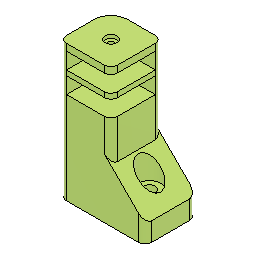
Idler Mount v18 (Autodesk Fusion 360 design; units mm, degrees)
Autodesk Fusion 360 part; units mm, degrees
note: some values were not read from the file. Chosen so that the rebuilt part matches the saved one: which face or edge a step refers to; which pieces of a blend or face edit are solid. Set by a fixed rule: which sketch regions a step uses.
box "BoxPrimitive1" add length 30 width 30 height 51.95 placed x (0, 0, 1) y (1, 0, 0) z (0, 1, 0) at (-10, 0, 0) makes body 1
box "BoxPrimitive2" add length 30 width 30 height 25.975 placed x (0, 0, 1) y (1, 0, 0) z (0, 1, 0) at (10, 0, 0) bodies 1
chamfer "Chamfer1" distance 20 angle 45 1 edges at (40, 25.975, 15) on bodies 1
sketch "Sketch3" plane through (0, 0, 0) normal (0, -1, 0) x (1, 0, 0)
  line L0 (40, 30) -> (-10, 30)
  line L1 (-10, 30) -> (-10, 0)
  line L2 (-10, 0) -> (40, 0)
  line L3 (40, 0) -> (40, 30)
  line L4 (0, 0) -> (20, 0) construction
  line L5 (19.9999, 30) -> (40, 30) construction
  line L6 (40, 30) -> (40, 0) construction
  line L7 (20, 0) -> (40, 0) construction
  line L8 (-10, 0) -> (-10, 30)
  line L9 (-10, 30) -> (40, 30)
  line L10 (-10, 0) -> (40, 0)
  line L11 (15, 30) -> (15, 0) construction
  line L12 (15, 0) -> (40, 30) construction
  line L13 (15, 30) -> (40, 0) construction
  circle A0 centre (27.5, 15) radius 3.5
move_body "Move1" bodies 1 to x (1, 0, 0) y (0, 1, 0) z (0, 0, 1) at (0, 5, 0)
extrude "Extrude1" add 1 faces at (6.6667, 5, 20) along direction (0, -1, 0) blind 5 on bodies 1 bodies 1
extrude "Extrude2" cut 1 faces at (10, 56.95, 10) along direction (0, -1, 0) blind 5 on bodies 1 bodies 1
fillet "Fillet1" radius 10 1 edges at (-10, 25.975, 0) on bodies 1
sketch "Sketch6" plane through (0, 51.95, 0) normal (0, 1, 0) x (-1, 0, 0)
  arc A0 (0, 0) -> (10, 10) centre (0, 10) ccw
  line L0 (10, 10) -> (10, 30)
  line L1 (10, 30) -> (-20, 30)
  line L2 (-20, 30) -> (-20, 0)
  line L3 (-20, 0) -> (0, 0)
  line L4 (-20, 0) -> (0, 0)
  line L5 (10, 30) -> (10, 10)
  line L6 (-20, 0) -> (-20, 30)
  line L7 (-20, 30) -> (10, 30)
  arc A1 (0, 0) -> (10, 10) centre (0, 10) ccw
  line L8 (10, 10) -> (10, 0)
  line L9 (10, 0) -> (0, 0)
  line L10 (10, 0) -> (-20, 30) construction
  line L11 (10, 30) -> (-20, 0) construction
  circle A2 centre (-5, 15) radius 1.5
  circle A3 centre (-5, 15) radius 11
  circle A4 centre (-5, 15) radius 2
  line L12 (-5, 15) -> (10, 15) construction
  line L13 (-5, 15) -> (-20, 15) construction
  line L14 (6, 15) -> (6, 30)
  line L15 (-5, 15) -> (-5, 4)
  line L16 (-5, 4) -> (-20, 4)
  line L17 (-16, 26) -> (-16, 30)
  line L18 (-16, 26) -> (-20, 26)
  line L19 (-16, 15) -> (-16, 26) construction
  line L20 (-5, 26) -> (-16, 26) construction
  dimension "d41" = 22
  measures "d41" diameter of A3
extrude "Extrude4" add 1 faces at (13.3333, 51.95, 10) along direction (0, 1, 0) blind 9 separate body on bodies 1 makes body 2
extrude "Extrude5" add 1 faces at (13.3333, 60.95, 10) along direction (0, 1, 0) blind 3 separate body on bodies 2 makes body 3
extrude "Extrude6" add 1 faces at (13.3333, 63.95, 10) along direction (0, 1, 0) blind 9 separate body on bodies 3 makes body 4
extrude "Extrude7" add 1 faces at (13.3333, 72.95, 10) along direction (0, 1, 0) blind 3 separate body on bodies 4 makes body 5
extrude "Extrude11" cut sketch "Sketch3" against normal blind 50 contours A0 bodies 1
sketch "Sketch10" plane through (0, 0, 0) normal (0, -1, 0) x (1, 0, 0)
  circle A0 centre (27.5, 15) radius 3.5
  arc A1 (-10, 10) -> (0, 0) centre (0, 10) ccw
  line L0 (0, 0) -> (40, 0)
  line L1 (40, 0) -> (40, 30)
  line L2 (40, 30) -> (-10, 30)
  line L3 (-10, 30) -> (-10, 10)
ref_plane "WorkPlane1" through (15, 15, 15) normal (0, -1, 0) x (1, 0, 0)
sketch "Sketch11" plane through (15, 15, 15) normal (0, -1, 0) x (1, 0, 0)
  circle A0 centre (12.5, 0) radius 3.5
  circle A1 centre (12.5, 0) radius 3.5
  line L0 (12.5, 0) -> (12.476, -3.4999)
cylinder "CylinderPrimitive4" cut diameter 13 height -21 placed x (1, 0, 0) y (0, 0, 1) z (0, -1, 0) at (27.5, 15, 15) bodies 1
extrude "Extrude12" cut sketch "Sketch6" along normal blind 38 contours A2 bodies 3 5
extrude "Extrude13" cut sketch "Sketch6" along normal blind 21 contours L1 L2 L6 L7 A3 L14 L16 L17 L18 | L1 L2 L6 L7 L17 L18 | A3 | A2 | A4 bodies 2 4
extrude "Extrude14" add sketch "Sketch6" along normal blind 24 contours L1 L2 L6 L7 L17 L18 bodies 3 2 1 5
sketch "Sketch12" plane through (0, 75.95, 0) normal (0, 1, 0) x (-1, 0, 0)
  circle A0 centre (-5, 15) radius 1.5
  line L0 (10, 30) -> (-20, 30)
  line L1 (-20, 30) -> (-20, 0)
  line L2 (-20, 0) -> (0, 0)
  arc A1 (0, 0) -> (10, 10) centre (0, 10) ccw
  line L3 (10, 10) -> (10, 30)
  line L4 (10, 30) -> (-20, 0) construction
  line L5 (-20, 30) -> (10, 0) construction
  line L6 (10, 0) -> (10, 30) construction
  line L7 (10, 0) -> (-20, 0) construction
  line L8 (-20, 0) -> (-20, 30) construction
  line L9 (-20, 30) -> (10, 30) construction
  circle A2 centre (-5, 15) radius 3.5
extrude "Extrude15" cut sketch "Sketch12" against normal blind 2 contours A2 bodies 3
extrude "Extrude16" add 1 faces at (4.9128, 75.95, 26.1634) along direction (0, 1, 0) blind 1 on bodies 3 bodies 3
extrude "Extrude17" add 1 faces at (2.1853, 73.95, 14.7516) along direction (0, 1, 0) blind 1 on bodies 3 bodies 3
extrude "Extrude18" cut sketch "Sketch6" against normal blind 8 contours A2 bodies 3
sketch "Sketch13" plane through (0, 63.95, 0) normal (0, 1, 0) x (-1, 0, 0)
  line L0 (-16, 26) -> (-20, 26)
  line L1 (-20, 26) -> (-20, 0)
  line L2 (-20, 0) -> (0, 0)
  arc A0 (0, 0) -> (10, 10) centre (0, 10) ccw
  line L3 (10, 10) -> (10, 30)
  line L4 (10, 30) -> (-16, 30)
  line L5 (-16, 30) -> (-16, 26)
  circle A1 centre (-5, 15) radius 1.5
  line L6 (10, 0) -> (-20, 30)
  line L7 (-20, 30) -> (10, 0) construction
  line L8 (10, 0) -> (10, 30) construction
  line L9 (-20, 0) -> (10, 0) construction
  line L10 (-20, 0) -> (10, 30) construction
  circle A2 centre (-5, 15) radius 1.5
  circle A3 centre (-5, 15) radius 2
extrude "Extrude19" add sketch "Sketch13" along normal blind 0.4 contours A1 L6 A2 A3 | A1 L6 A2 A3 bodies 3
extrude "Extrude20" add sketch "Sketch6" along normal blind 0.4 contours A4 bodies 3
extrude "Extrude21" cut 1 faces at (5, 52.35, 13.1704) along direction (0, -1, 0) blind 0.2 on bodies 3 bodies 3
extrude "Extrude22" cut 1 faces at (3.1797, 64.35, 14.8261) along direction (0, -1, 0) blind 0.2 on bodies 3 bodies 3
extrude "Extrude23" add sketch "Sketch13" against normal blind 3.2 contours A1 L6 A2 A3 | A1 L6 A2 A3 bodies 3
sketch "Sketch14" plane through (0, 72.95, 0) normal (0, -1, 0) x (1, 0, 0)
  line L0 (20, 26) -> (16, 26)
  line L1 (16, 26) -> (16, 30)
  line L2 (16, 30) -> (-10, 30)
  line L3 (-10, 30) -> (-10, 10)
  arc A0 (-10, 10) -> (0, 0) centre (0, 10) ccw
  line L4 (0, 0) -> (20, 0)
  line L5 (20, 0) -> (20, 26)
  circle A1 centre (5, 15) radius 1.5
  circle A2 centre (5, 15) radius 1.5
  circle A3 centre (5, 15) radius 2
extrude "Extrude24" add sketch "Sketch14" along normal blind 0.2 contours A3 bodies 3
combine "Combine1" operation add target body 2 tool bodies 3 4
fillet "Fillet2" radius 4 1 edges at (-10, 38.475, 30) on bodies 2
fillet "Fillet3" radius 4 1 edges at (20, 53.9625, 30) on bodies 2
fillet "Fillet4" radius 4 1 edges at (20, 53.9625, 0) on bodies 2
fillet "Fillet5" radius 4 2 edges at (40, 5.4875, 0) (40, 5.4875, 30) on bodies 2
ref_plane "WorkPlane2" through (5, 47.95, 15) normal (0, 1, 0) x (-1, 0, 0)
split "Split1" by plane through (5, 47.95, 15) normal (0, 1, 0) bodies 2 makes body 6 at (16.1667, 76.95, 15)
extrude "Extrude25" cut 1 faces at (17.3333, 66.95, 26) along direction (0, 0, 1) blind 12 on bodies 6 bodies 6
extrude "Extrude26" cut 1 faces at (18.6667, 54.95, 26) along direction (0, 0, 1) blind 15 on bodies 6 bodies 6
extrude "Extrude38" cut 1 faces at (3.1797, 64.15, 14.8261) along direction (0, -1, 0) blind 0.5 on bodies 6 bodies 6
extrude "Extrude39" cut 1 faces at (5.0684, 63.95, 25.6648) along direction (0, -1, 0) blind 0.5 on bodies 6 bodies 6
extrude "Extrude40" add 1 faces at (5.0684, 60.95, 25.6648) along direction (0, -1, 0) blind 0.5 on bodies 6 bodies 6
extrude "Extrude41" add 1 faces at (3.1797, 60.75, 15.1739) along direction (0, -1, 0) blind 0.5 on bodies 6 bodies 6
extrude "Extrude42" cut 1 faces at (5.0684, 51.95, 25.6648) along direction (0, -1, 0) blind 1 on bodies 6 bodies 6
extrude "Extrude43" cut 1 faces at (3.1797, 52.15, 15.1739) along direction (0, -1, 0) blind 1 on bodies 6 bodies 6
extrude "Extrude44" add 1 faces at (3.1797, 51.15, 15.1739) along direction (0, 1, 0) blind 0.1 on bodies 6 bodies 6
extrude "Extrude45" add 1 faces at (3.1797, 60.25, 15.1739) along direction (0, -1, 0) blind 0.1 on bodies 6 bodies 6
extrude "Extrude46" add 1 faces at (6.8203, 72.75, 14.8261) along direction (0, -1, 0) blind 0.1 on bodies 6 bodies 6
extrude "Extrude47" add 1 faces at (3.1797, 63.65, 14.8261) along direction (0, 1, 0) blind 0.1 on bodies 6 bodies 6
fillet "Fillet9" radius 2.5 1 edges at (6.8647, 63.45, 14.2768) on bodies 6
fillet "Fillet10" radius 2.5 3 edges at (6.8647, 60.45, 14.2768) (6.8647, 50.95, 14.2768) (3.1353, 72.95, 15.7232) on bodies 6
move_body "Move4" bodies 6 to x (1, 0, 0) y (0, 1, 0) z (0, 0, 1) at (0, 3, 0)
extrude "Extrude59" add 1 faces at (15.5, 50.95, 15) along direction (0, -1, 0) blind 3 on bodies 6 bodies 6 2
copy_body "Body->Comp2" bodies 6 removing the originals makes body 7 in component "Idler Mount"
component "Idler Mount" placed x (1, 0, 0) y (0, 1, 0) z (0, 0, 1) at (0, 0, 0)
equation "d8 = 51.95 mm / 2"
equation "d57 = 22 mm - 30 mm"
equation "d67 = -3.00 mm - 0.2 mm"
